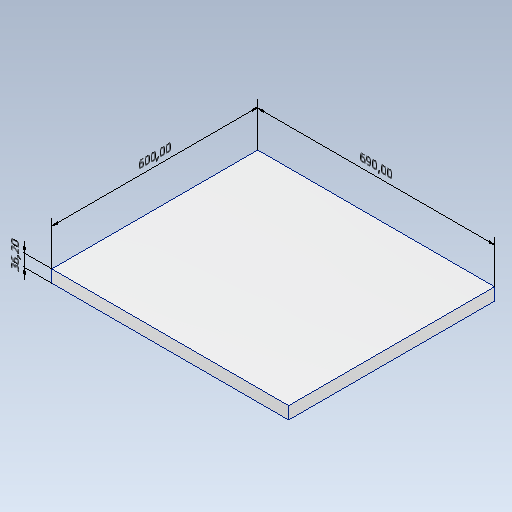
# Autodesk Inventor part: piso2
Saved by Autodesk Inventor 2021 (Build 250183000, 183)
## iProperties
Created: 2020-10-29
Part Number: piso2
Material: Aluminio 6061
Document SubType Name: Modeling
Designer: germi
Density: 2.7 g/cm^3
Appearance: Aluminio - Plano
Mass: 40464.4 g
Surface Area: 9213.96 cm^2
Volume: 14986.8 cm^3
Author: germi
Autodesk Inventor part; units mm, degrees
ref_plane "YZ Plane" through (0, 0, 0) normal (1, 0, 0) x (0, 1, 0)
ref_plane "XZ Plane" through (0, 0, 0) normal (0, 1, 0) x (-1, 0, 0)
ref_plane "XY Plane" through (0, 0, 0) normal (0, 0, 1) x (1, 0, 0)
sketch "Boceto1" plane through (0, 0, 0) normal (0, 1, 0) x (-1, 0, 0)
  line L0 (-690, 0) -> (-690, -628.4316)
  line L1 (0, -628.4316) -> (0, 0)
  line L2 (0, 0) -> (-260, 0)
  line L3 (-430, 0) -> (-690, 0)
  line L4 (-690, -600) -> (-430, -600)
  line L5 (-260, -600) -> (0, -600)
  line L6 (-260, -600) -> (-430, -600)
  line L7 (-430, 0) -> (-260, 0)
  point P0 (0, -600)
  dimension "d16" = 690
  dimension "d21" = 600
  dimension "d22" = 600
  constraints: 16 end point, 5 parallel, 2 horizontal, 2 perpendicular, 1 collinear
  measures "d16" distance between parallel lines of L0 L1
  measures "d21" distance between parallel lines of L5 L2
  measures "d22" distance between parallel lines of L4 L3
extrude "Extrusión1" add sketch "Boceto1" along normal blind 36.2
